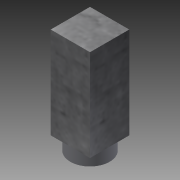
# Autodesk Inventor part: EF-Arm
Saved by Autodesk Inventor 2015 (Build 190159000, 159)
## iProperties
Created: 2016-12-02
Part Number: EF-Arm
Material: Generic
Document SubType Name: Modeling
Designer: Ernest
Density: 1 g/cm^3
Appearance: Default
Author: Ernest
Autodesk Inventor part; units mm, degrees
ref_plane "YZ Plane" through (0, 0, 0) normal (1, 0, 0) x (0, 1, 0)
ref_plane "XZ Plane" through (0, 0, 0) normal (0, 1, 0) x (-1, 0, 0)
ref_plane "XY Plane" through (0, 0, 0) normal (0, 0, 1) x (1, 0, 0)
sketch "Sketch1" plane through (0, 0, 0) normal (0, 0, 1) x (1, 0, 0)
  line L0 (0, 0) -> (15, 0)
  line L1 (15, 0) -> (15, 15)
  line L2 (15, 15) -> (0, 15)
  line L3 (0, 15) -> (0, 0)
  dimension "d0" = 15
  dimension "d1" = 15
  constraints: 8 end point, 2 parallel, 1 horizontal, 1 perpendicular
  measures "d0" distance of L2.end L1.end
  measures "d1" distance of L1.end L0.end
extrude "Extrusion1" add sketch "Sketch1" along normal blind 40
sketch "Sketch2" plane through (0, 0, 0) normal (0, 0, -1) x (-1, 0, 0)
  circle A0 centre (-7.5, 7.5) radius 7.5
  line L0 (-15, 15) -> (0, 15)
  line L1 (0, 15) -> (0, 0)
  line L2 (0, 0) -> (-15, 0)
  line L3 (-15, 0) -> (-15, 15)
  line L4 (-15, 15) -> (0, 15) projected
  line L5 (0, 0) -> (-15, 0) projected
  line L6 (0, 15) -> (0, 0) projected
  line L7 (-15, 0) -> (-15, 15) projected
  constraints: 8 end point, 4 tangent, 2 parallel, 1 centre point, 1 horizontal, 1 perpendicular
extrude "Extrusion2" cut sketch "Sketch2" against normal blind 5 contours L1 L2 A0 | A0 L0 L1 | A0 L3 L0 | L2 L3 A0
body "Solid1"
